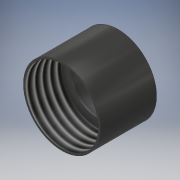
# Autodesk Inventor part: Tutup lampu
Saved by Autodesk Inventor 2019.5 (Build 235369000, 369)
## iProperties
Created: 2022-10-11
Part Number: Tutup lampu
Material: Aluminum 6061-AHC
Document SubType Name: Modeling
Designer: ASUS
Density: 2.7 g/cm^3
Appearance: Aluminum - Dark
Author: ASUS
Autodesk Inventor part; units mm, degrees
ref_plane "YZ Plane" through (0, 0, 0) normal (1, 0, 0) x (0, 1, 0)
ref_plane "XZ Plane" through (0, 0, 0) normal (0, 1, 0) x (-1, 0, 0)
ref_plane "XY Plane" through (0, 0, 0) normal (0, 0, 1) x (1, 0, 0)
sketch "Sketch1" plane through (0, 0, 0) normal (0, 0, 1) x (1, 0, 0)
  circle A0 centre (0, 0) radius 20.5
  dimension "d0" = 41
  constraints: 1 centre point, 1 coincident
  measures "d0" diameter of A0
extrude "Extrusion1" add sketch "Sketch1" along normal blind 30
sketch "Sketch2" plane through (0, 0, 0) normal (0, 0, -1) x (-1, 0, 0)
  point P0 (0, 0)
  point P1 (0, 0)
  constraints: 1 coincident
hole "Hole1" at (0, 0, 0) direction (0, 0, 1) diameter 37 depth 10
shell "Shell1" thickness 1 removed faces 1 at (3.5154, 4.1371, 30)
thread "Thread1" size "M39x4" class "6H" standard "ANSI Metric M Profile" full length
sketch "Sketch4" plane through (0, 0, 10) normal (0, 0, -1) x (-1, 0, 0)
  point P0 (0, 0)
  point P1 (0, 0)
  constraints: 1 coincident
hole "Hole2" at (0, 0, 10) direction (0, 0, 1) diameter 30 depth 30
body "Solid1"
